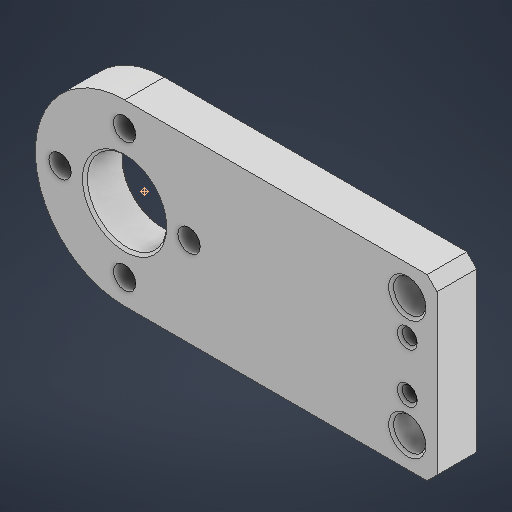
# Autodesk Inventor part: Support
Saved by Autodesk Inventor 2025.4 (Build 294407000, 407)
## iProperties
Created: 2026-05-29
Part Number: Support
Material: Generic
Document SubType Name: Modeling
Designer: VuQuan
Density: 1 g/cm^3
Appearance: Default
Author: VuQuan
Autodesk Inventor part; units mm, degrees
ref_plane "YZ Plane" through (0, 0, 0) normal (1, 0, 0) x (0, 1, 0)
ref_plane "XZ Plane" through (0, 0, 0) normal (0, 1, 0) x (-1, 0, 0)
ref_plane "XY Plane" through (0, 0, 0) normal (0, 0, 1) x (1, 0, 0)
sketch "Sketch1" plane through (0, 0, 0) normal (0, 0, 1) x (1, 0, 0)
  circle A0 centre (0, 0) radius 8
  circle A1 centre (0, 0) radius 13 construction
  line L0 (0, 18) -> (63, 18)
  line L1 (63, 18) -> (63, -18)
  line L2 (63, -18) -> (0, -18)
  arc A2 (0, 18) -> (0, -18) centre (0, 0) ccw
  circle A3 centre (0, 13) radius 2.25
  circle A4 centre (-13, 0) radius 2.25
  circle A5 centre (0, -13) radius 2.25
  circle A6 centre (13, 0) radius 2.25
  line L3 (63, 0) -> (0, 0) construction
  circle A7 centre (57, 5) radius 1.5
  circle A8 centre (57, 12) radius 3.25
  circle A9 centre (57, -5) radius 1.5
  circle A10 centre (57, -12) radius 3.25
  dimension "d1" = 26
  dimension "d0" = 16
  dimension "d2" = 63
  dimension "d3" = 18
  dimension "d4" = 4.5
  dimension "d7" = 360
  dimension "d9" = 3
  dimension "d10" = 6.5
  dimension "d11" = 10
  dimension "d12" = 24
  dimension "d13" = 57
  constraints: 10 centre point, 8 end point, 3 coincident, 3 vertical alignment, 2 horizontal, 2 perpendicular, 2 point on circle, 2 symmetric about line, 2 tangent, 1 midpoint, 13 other
  measures "d0" diameter of A0
  measures "d2" distance from line of L1 point (0, 0)
  measures "d3" radius of A2
  measures "d4" diameter of A3
  measures "d9" diameter of A7
  measures "d10" diameter of A8
  measures "d11" diameter of A7.centre L3
  measures "d12" diameter of A8.centre L3
  measures "d13" horizontal distance of A8.centre point (0, 0)
extrude "Extrusion1" add sketch "Sketch1" along normal mid plane 8
chamfer "Chamfer1" distance 0.5 angle 45 10 edges at (-8, 0, 4) (-8, 0, -4) (53.75, -12, 4) (53.75, -12, -4) (55.5, -5, 4) (55.5, -5, -4) (55.5, 5, -4) (55.5, 5, 4) (53.75, 12, 4) (53.75, 12, -4)
chamfer "Chamfer2" distance 2 angle 45 2 edges at (63, 18, 0) (63, -18, 0)
body "Solid1"
